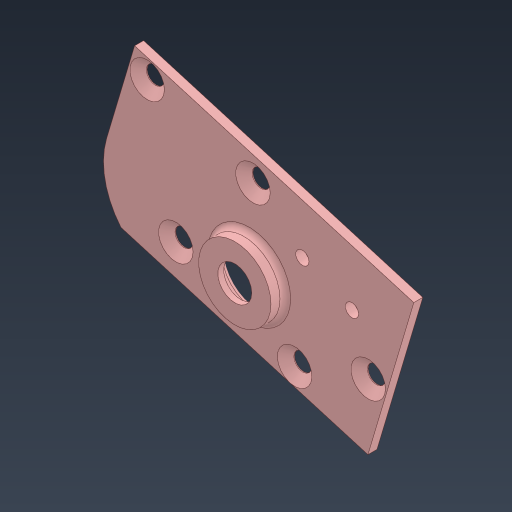
# Autodesk Inventor part: gearbox-right-wall
Saved by Autodesk Inventor 2023 (Build 270158000, 158)
## iProperties
Created: 2025-04-29
Part Number: gearbox-right-wall
Material: Generic
Document SubType Name: Modeling
Designer: szymo
Density: 1 g/cm^3
Appearance: Default(1)
Mass: 2.94866 g
Surface Area: 35.4918 cm^2
Volume: 2.94866 cm^3
Author: szymo
Autodesk Inventor part; units mm, degrees
ref_plane "YZ Plane" through (0, 0, 0) normal (1, 0, 0) x (0, 1, 0)
ref_plane "XZ Plane" through (0, 0, 0) normal (0, 1, 0) x (-1, 0, 0)
ref_plane "XY Plane" through (0, 0, 0) normal (0, 0, 1) x (1, 0, 0)
ref_plane "Work Plane1" through (0, 0, 0) normal (0, 0, 1) x (1, 0, 0)
ref_plane "Work Plane2" through (-12.3348, -13.8221, 0.7) normal (0, 0, 1) x (0.8864221, 0.4628777, 0)
sketch "Sketch1" plane through (0, 0, 0) normal (0, 0, 1) x (1, 0, 0)
  circle A0 centre (-15.5866, -4.8003) radius 2.75 projected
  circle A1 centre (6.7658, -13.901) radius 2.75 projected
  circle A2 centre (-1.0723, 12.0762) radius 2.75 projected
  circle A3 centre (20.6128, -9.0349) radius 2.75 projected
  circle A4 centre (12.5717, -14.649) radius 2.25 projected
  line L0 (20.5612, -21.3803) -> (29.1927, 7.7091) projected
  line L1 (29.1927, 7.7091) -> (-23.3434, 23.2977) projected
  line L2 (-23.3434, 23.2977) -> (-28.6039, 5.5687) projected
  arc A5 (-28.6039, 5.5687) -> (-25.9011, -7.5939) centre (-14.9427, 1.5151) ccw projected
  line L3 (-25.9011, -7.5939) -> (20.5612, -21.3803) projected
  arc A6 (0.0711, 6.5509) -> (7.2487, -7.558) centre (-1.7876, -3.2749) ccw projected
  circle A7 centre (-1.7876, -3.2749) radius 6 projected
  circle A8 centre (-1.7876, -3.2749) radius 6
  arc A9 (7.2487, -7.558) -> (17.9688, -6.473) centre (12.5717, -6.649) ccw projected
  arc A10 (16.0276, 7.6501) -> (0.0711, 6.5509) centre (8.226, 4.5365) ccw projected
  arc A11 (17.9688, -6.473) -> (16.0276, 7.6501) centre (17.5545, 0.665) ccw projected
  point P0 (0, 0)
  dimension "d25" = 12
  constraints: 1 centre point
  measures "d25" diameter of A8
extrude "Extrusion1" add sketch "Sketch1" along normal up to surface (0.7 mm away) contours A0 | A1 | A2 | A3 | A4 | L3 A5 L2 L1 L0 | A10 A11 A9 A6
sketch "Sketch2" plane through (0, 0, 0.7) normal (0, 0, 1) x (1, 0, 0)
  line L0 (29.1927, 7.7091) -> (-23.3434, 23.2977) projected
  line L1 (-23.3434, 23.2977) -> (-28.6039, 5.5687) projected
  arc A0 (-28.6039, 5.5687) -> (-25.9011, -7.5939) centre (-14.9427, 1.5151) ccw projected
  line L2 (-25.9011, -7.5939) -> (20.5612, -21.3803) projected
  line L3 (20.5612, -21.3803) -> (29.1927, 7.7091) projected
  circle A1 centre (-1.7876, -3.2749) radius 6.3 projected
  circle A2 centre (-1.7876, -3.2749) radius 4 projected
  circle A3 centre (-1.7876, -3.2749) radius 6
  point P0 (0, 0)
  dimension "d26" = 12
  constraints: 1 centre point
  measures "d26" diameter of A3
extrude "Extrusion2" add sketch "Sketch2" along normal blind 1 contours L3 L2 A0 L1 L0 | A1
sketch "Sketch3" plane through (0, 0, 1.7) normal (0, 0, 1) x (1, 0, 0)
  circle A0 centre (-15.5866, -4.8003) radius 2.75 projected
  circle A1 centre (6.7658, -13.901) radius 2.75 projected
  circle A2 centre (-1.0723, 12.0762) radius 2.75 projected
  circle A3 centre (20.6128, -9.0349) radius 2.75 projected
  circle A4 centre (12.5717, -14.649) radius 2.25 projected
  line L0 (20.5612, -21.3803) -> (29.1927, 7.7091) projected
  line L1 (29.1927, 7.7091) -> (-23.3434, 23.2977) projected
  line L2 (-23.3434, 23.2977) -> (-28.6039, 5.5687) projected
  arc A5 (-28.6039, 5.5687) -> (-25.9011, -7.5939) centre (-14.9427, 1.5151) ccw projected
  line L3 (-25.9011, -7.5939) -> (20.5612, -21.3803) projected
  arc A6 (0.0711, 6.5509) -> (7.2487, -7.558) centre (-1.7876, -3.2749) ccw projected
  arc A7 (7.2487, -7.558) -> (17.9688, -6.473) centre (12.5717, -6.649) ccw projected
  arc A8 (16.0276, 7.6501) -> (0.0711, 6.5509) centre (8.226, 4.5365) ccw projected
  arc A9 (17.9688, -6.473) -> (16.0276, 7.6501) centre (17.5545, 0.665) ccw projected
  circle A10 centre (-20.9836, 18.9466) radius 2.75 projected
  point P0 (0, 0)
  point P1 (-1.0723, 12.0762)
  point P2 (-15.5866, -4.8003)
  point P3 (6.7658, -13.901)
  point P4 (20.6128, -9.0349)
  constraints: 5 coincident
hole "Hole1" at (-1.0723, 12.0762, 1.7) at (-15.5866, -4.8003, 1.7) at (6.7658, -13.901, 1.7) at (20.6128, -9.0349, 1.7) at (-20.9836, 18.9466, 1.7) direction (0, 0, -1) diameter 3.4 depth 5 countersink diameter 6.5 countersink angle 90 clearance for "Countersunk Flat Head Screw ISO 2009/7046" size "M3" standard "ISO"
sketch "Sketch4" plane through (0, 0, 0) normal (0, 0, -1) x (-1, 0, 0)
  circle A0 centre (-8.226, 4.5365) radius 1.25 projected
  circle A1 centre (-17.5545, 0.665) radius 1.25 projected
  circle A2 centre (-17.5545, 0.665) radius 1.25
  circle A3 centre (-8.226, 4.5365) radius 1.25
  point P0 (0, 0)
  dimension "d20" = 0
  dimension "d21" = 0
  constraints: 2 centre point
  measures "d20" radial gap between concentric circles of A0 A3
  measures "d21" radial gap between concentric circles of A2 A1
extrude "Extrusion3" cut sketch "Sketch4" against normal blind 7.75
sketch "Sketch7" plane through (0, 0, 1.7) normal (0, 0, 1) x (1, 0, 0)
  circle A0 centre (-1.7876, -3.2749) radius 6 projected
  arc A1 (5.9967, -17.0587) -> (5.6882, -16.9671) centre (6.7658, -13.901) ccw projected
  line L0 (5.9967, -17.0587) -> (20.5612, -21.3803) projected
  line L1 (20.5612, -21.3803) -> (29.1927, 7.7091) projected
  circle A2 centre (20.6128, -9.0349) radius 3.25 projected
  line L2 (29.1927, 7.7091) -> (-23.3434, 23.2977) projected
  line L3 (-23.3434, 23.2977) -> (-28.6039, 5.5687) projected
  arc A3 (-28.6039, 5.5687) -> (-25.9011, -7.5939) centre (-14.9427, 1.5151) ccw projected
  line L4 (-25.9011, -7.5939) -> (5.6882, -16.9671) projected
  circle A4 centre (-15.5866, -4.8003) radius 3.25 projected
  circle A5 centre (-1.0723, 12.0762) radius 3.25 projected
  circle A6 centre (-1.7876, -3.2749) radius 6 projected
  circle A7 centre (-1.7876, -3.2749) radius 6.8
  point P0 (0, 0)
  dimension "d27" = 0.8
  constraints: 1 centre point
  measures "d27" radial gap between concentric circles of A0 A7
extrude "Extrusion6" add sketch "Sketch7" along normal blind 1.6 contours A7
sketch "Sketch8" plane through (-1.7876, -3.2749, 3.3) normal (0, 0, 1) x (1, 0, 0)
  circle A0 centre (0, 0) radius 6.8 projected
  circle A1 centre (0, 0) radius 3.2
  point P0 (1.7876, 3.2749)
  dimension "d30" = 6.4
  constraints: 1 centre point, 1 coincident
  measures "d30" diameter of A1
extrude "Extrusion7" add sketch "Sketch8" along normal blind 1.1
fillet "Fillet4" radius 1 1 edges at (-8.5876, -3.2749, 1.7)
fillet "Fillet6" radius 0.8 1 edges at (-7.7876, -3.2749, 0)
sketch "Sketch9" plane through (8.226, 4.5365, 1.5) normal (0, 0, -1) x (-1, 0, 0)
  circle A0 centre (-9.3285, -3.8715) radius 1.55 projected
  circle A1 centre (0, 0) radius 1.55 projected
  point P0 (8.226, -4.5365)
extrude "Extrusion8" [suppressed]
body "Solid1"
